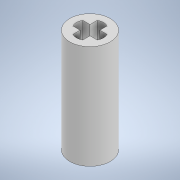
# Autodesk Inventor part: motor_adapt
Saved by Autodesk Inventor 2021 (Build 250183000, 183)
## iProperties
Created: 2024-04-09
Part Number: motor_adapt
Material: Generic
Document SubType Name: Modeling
Designer: 23adrdam
Density: 1 g/cm^3
Appearance: Default
Author: 23adrdam
Autodesk Inventor part; units mm, degrees
ref_plane "YZ Plane" through (0, 0, 0) normal (1, 0, 0) x (0, 1, 0)
ref_plane "XZ Plane" through (0, 0, 0) normal (0, 1, 0) x (-1, 0, 0)
ref_plane "XY Plane" through (0, 0, 0) normal (0, 0, 1) x (1, 0, 0)
sketch "Sketch3" plane through (0, 0, 0) normal (0, 1, 0) x (-1, 0, 0)
  line L0 (2.3926, -0.9756) -> (2.3926, 0.9756)
  line L1 (2.3926, 0.9756) -> (0.9755, 0.9755)
  line L2 (0.9755, 0.9755) -> (0.9754, 2.3926)
  line L3 (0.9754, 2.3926) -> (-0.9756, 2.3926)
  arc A0 (0.9754, 2.3926) -> (-0.9756, 2.3926) centre (0, 0.8054) ccw
  arc A1 (2.3926, -0.9756) -> (2.3926, 0.9756) centre (0.8054, 0) ccw
  line L4 (2.3926, -0.9756) -> (0.9755, -0.9756)
  line L5 (0.9755, -0.9756) -> (0.9756, -2.3926)
  line L6 (0.9756, -2.3926) -> (-0.9755, -2.3926)
  arc A2 (-0.9755, -2.3926) -> (0.9756, -2.3926) centre (0, -0.8054) ccw
  line L7 (-0.9756, 2.3926) -> (-0.9756, 0.9756)
  line L8 (-0.9755, -2.3926) -> (-0.9756, -0.9755)
  line L9 (-0.9756, 0.9756) -> (-2.3926, 0.9756)
  line L10 (-2.3926, 0.9756) -> (-2.3925, -0.9755)
  line L11 (-2.3925, -0.9755) -> (-0.9756, -0.9755)
  arc A3 (-2.3926, 0.9756) -> (-2.3925, -0.9755) centre (-0.8054, 0) ccw
  circle A4 centre (0, 0) radius 4
  dimension "d23" = 1.951
  dimension "d24" = 1.9511
  dimension "d25" = 0.9756
  dimension "d28" = 1.4171
  dimension "d29" = 1.417
  dimension "d30" = 2.5838
  dimension "d31" = 1.863
  dimension "d32" = 1.863
  dimension "d33" = 1.417
  dimension "d34" = 1.9511
  dimension "d35" = 1.863
  dimension "d36" = 1.417
  dimension "d37" = 2.5838
  dimension "d38" = 1.9511
  dimension "d39" = 1.863
  dimension "d40" = 2.3925
  dimension "d41" = 2.3925
  dimension "d42" = 1.417
  dimension "d43" = 1.417
  dimension "d44" = 8
  constraints: 24 end point, 8 point on circle, 7 perpendicular, 6 coincident, 5 centre point, 2 horizontal, 2 vertical
  measures "d23" distance of L2.end L3.end
  measures "d24" distance of L0.start L0.end
  measures "d25" vertical distance of point (0, 0) L0.start
  measures "d28" distance of L0.end L1.end
  measures "d29" distance of L1.end L2.end
  measures "d30" distance of L0.start point (0, 0)
  measures "d31" radius of A0
  measures "d32" radius of A1
  measures "d33" distance of L4.end L5.end
  measures "d34" distance of L5.end L6.end
  measures "d35" radius of A2
  measures "d36" distance of L0.start L4.end
  measures "d37" distance of L10.end point (0, 0)
  measures "d38" distance of L9.end L10.end
  measures "d39" radius of A3
  measures "d40" distance from line of L3 point (0, 0)
  measures "d41" distance from line of L10 point (0, 0)
  measures "d42" distance of L7.end L9.end
  measures "d43" distance of L6.end L8.end
  measures "d44" diameter of A4
extrude "Extrusion1" add sketch "Sketch3" along normal blind 10
sketch "Sketch4" plane through (0, 0, 0) normal (0, -1, 0) x (1, 0, 0)
  circle A0 centre (0, 0) radius 4
  constraints: 1 centre point, 1 coincident
extrude "Extrusion2" add sketch "Sketch4" along normal blind 0.5
sketch "Sketch5" plane through (0, -0.5, 0) normal (0, -1, 0) x (1, 0, 0)
  circle A0 centre (0, 0) radius 2.8975
  line L0 (0, 1.9675) -> (-2.1271, 1.9675)
  line L1 (-0.9754, 2.3926) -> (-0.9755, 0.9755) projected
  line L2 (0, 1.9675) -> (2.1271, 1.9675)
  line L3 (0, -1.968) -> (-2.1267, -1.968)
  line L4 (-0.9755, -0.9756) -> (-0.9756, -2.3926) projected
  line L5 (0, -1.968) -> (2.1267, -1.968)
  circle A1 centre (0, 0) radius 4
  dimension "d49" = 5.795
  dimension "d50" = 1.9675
  dimension "d51" = 1.968
  dimension "d52" = 2.1271
  dimension "d53" = 2.1267
  dimension "d56" = 8
  constraints: 8 end point, 4 point on circle, 2 centre point, 2 perpendicular, 1 coincident, 1 horizontal, 1 point on line
  measures "d49" diameter of A0
  measures "d50" distance of A0.centre L0.start
  measures "d51" distance of A0.centre L3.start
  measures "d52" distance of L0.start L0.end
  measures "d53" distance of L3.start L5.end
  measures "d56" diameter of A1
extrude "Extrusion3" add sketch "Sketch5" along normal blind 10 contours L2 L0 A0 | A0 L3 L5 | A1
body "Solid1"
